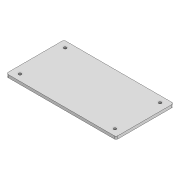
# Autodesk Inventor part: Spacer
Saved by Autodesk Inventor 2020 (Build 240168000, 168)
## iProperties
Created: 2020-11-07
Part Number: Spacer
Material: Generic
Document SubType Name: Modeling
Designer: ferrerx
Density: 1 g/cm^3
Appearance: Default
Author: ferrerx
Autodesk Inventor part; units mm, degrees
ref_plane "YZ Plane" through (0, 0, 0) normal (1, 0, 0) x (0, 1, 0)
ref_plane "XZ Plane" through (0, 0, 0) normal (0, 1, 0) x (-1, 0, 0)
ref_plane "XY Plane" through (0, 0, 0) normal (0, 0, 1) x (1, 0, 0)
sketch "Sketch1" plane through (0, 0, 0) normal (0, 1, 0) x (-1, 0, 0)
  line L0 (0, 0) -> (150, 0)
  line L1 (150, 0) -> (150, -140)
  line L2 (150, -140) -> (0, -140)
  line L3 (0, -140) -> (0, 0)
  line L4 (150, -70) -> (0, -70) construction
  line L5 (24, -45.75) -> (126, -45.75) construction
  line L6 (126, -45.75) -> (126, -94.25) construction
  line L7 (126, -94.25) -> (24, -94.25) construction
  line L8 (24, -94.25) -> (24, -45.75) construction
  line L9 (24, -45.75) -> (126, -94.25) construction
  line L10 (126, -45.75) -> (24, -94.25) construction
  circle A0 centre (126, -45.75) radius 1.5
  circle A1 centre (126, -94.25) radius 1.5
  circle A2 centre (24, -94.25) radius 1.5
  circle A3 centre (24, -45.75) radius 1.5
  point P0 (75, -70)
  dimension "d0" = 150
  dimension "d1" = 140
  dimension "d2" = 102
  dimension "d3" = 48.5
  dimension "d4" = 3
  dimension "d5" = 3
  dimension "d6" = 3
  dimension "d7" = 3
  constraints: 22 end point, 5 midpoint, 4 centre point, 4 coincident, 4 parallel, 2 horizontal, 2 perpendicular
  measures "d0" distance of L1.end L2.end
  measures "d1" distance of L0.end L1.end
  measures "d2" distance of L6.end L7.end
  measures "d3" distance of L7.end L5.start
  measures "d4" diameter of A1
  measures "d5" diameter of A0
  measures "d6" diameter of A3
  measures "d7" diameter of A2
extrude "Extrusion1" add sketch "Sketch1" along normal blind 3
sketch "Sketch2" plane through (0, 3, 0) normal (0, 1, 0) x (1, 0, 0)
  line L0 (-150, 140) -> (-150, 0) projected
  line L1 (-150, 50) -> (-147, 50)
  line L2 (-147, 50) -> (-147, 90)
  line L3 (-147, 90) -> (-150, 90)
  line L4 (-150, 90) -> (-150, 50)
  line L5 (-147, 70) -> (-150, 70) construction
  line L6 (0, 0) -> (0, 140) projected
  line L7 (0, 70) -> (-150, 70) construction
  line L8 (-150, 0) -> (0, 0) projected
  line L9 (-75, 0) -> (-75, 98) construction
  line L10 (-95, 0) -> (-55, 0)
  line L11 (-55, 0) -> (-55, 3)
  line L12 (-55, 3) -> (-95, 3)
  line L13 (-95, 3) -> (-95, 0)
  line L14 (-75, 3) -> (-75, 0) construction
  line L15 (0, 50) -> (-3, 50)
  line L16 (-3, 50) -> (-3, 90)
  line L17 (-3, 90) -> (0, 90)
  line L18 (0, 90) -> (0, 50)
  line L19 (-3, 70) -> (0, 70) construction
  line L20 (-95, 140) -> (-55, 140)
  line L21 (-55, 140) -> (-55, 137)
  line L22 (-55, 137) -> (-95, 137)
  line L23 (-95, 137) -> (-95, 140)
  line L24 (-75, 137) -> (-75, 140) construction
  point P0 (0, 50)
  point P1 (0, 90)
  point P2 (-55, 0)
  dimension "d10" = 40
  dimension "d11" = 3
  dimension "d12" = 40
  dimension "d13" = 3
  constraints: 44 end point, 14 symmetric about line, 7 midpoint, 4 parallel, 3 perpendicular, 2 collinear, 2 horizontal, 2 point on line, 1 vertical
  measures "d10" distance of L1.end L2.end
  measures "d11" distance of L2.end L3.end
  measures "d12" distance between parallel lines of L11 L13
  measures "d13" distance of L10.end L11.end
extrude "Extrusion2" cut sketch "Sketch2" against normal blind 5
sketch "Sketch3" plane through (0, 3, 0) normal (0, 1, 0) x (1, 0, 0)
  line L0 (-147, 50) -> (-147, 90) projected
  line L1 (-147, 70) -> (-3, 70) construction
  line L2 (-3, 50) -> (-3, 90) projected
  line L3 (-134, 39) -> (-16, 39)
  line L4 (-16, 39) -> (-16, 101)
  line L5 (-16, 101) -> (-134, 101)
  line L6 (-134, 101) -> (-134, 39)
  line L7 (-134, 39) -> (-16, 101) construction
  line L8 (-16, 39) -> (-134, 101) construction
  point P0 (0, 0)
  point P1 (-75, 70)
  dimension "d16" = 118
  dimension "d17" = 62
  constraints: 14 end point, 5 midpoint, 2 parallel, 1 horizontal, 1 perpendicular
  measures "d16" distance of L3.start L3.end
  measures "d17" distance of L3.end L4.end
extrude "Extrusion3" cut sketch "Sketch3" against normal blind 10 keep common part
fillet "Fillet1" radius 2 4 edges at (-16, 1.5, -39) (-16, 1.5, -101) (-134, 1.5, -39) (-134, 1.5, -101)
body "Solid1"
